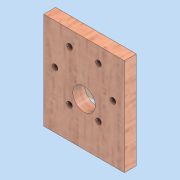
# Autodesk Inventor part: Motor
Saved by Autodesk Inventor 2021 (Build 250183000, 183)
## iProperties
Created: 2021-02-01
Part Number: Motor
Material: Generic
Document SubType Name: Modeling
Designer: garre
Density: 1 g/cm^3
Appearance: Default
Author: garre
Autodesk Inventor part; units mm, degrees
ref_plane "YZ Plane" through (0, 0, 0) normal (1, 0, 0) x (0, 1, 0)
ref_plane "XZ Plane" through (0, 0, 0) normal (0, 1, 0) x (-1, 0, 0)
ref_plane "XY Plane" through (0, 0, 0) normal (0, 0, 1) x (1, 0, 0)
sketch "Sketch1" plane through (0, 0, 0) normal (0, 0, 1) x (1, 0, 0)
  point P0 (0, 0)
ref_plane "Work Plane1" through (0, 0, 0) normal (0, 0, 1) x (1, 0, 0)
sketch "Sketch5" plane through (0, 0, 0) normal (0, 0, 1) x (1, 0, 0)
  circle A0 centre (-15.5, 0) radius 1.5
  circle A1 centre (0, 0) radius 18.4 projected
  line L0 (-18.4, 0) -> (18.4, 0)
  line L1 (-1.5961, -18.3306) -> (-1.5961, -18.3306)
  line L2 (0, 18.4) -> (0, -18.4)
  circle A2 centre (0, -7) radius 6
  circle A3 centre (15.5, 0) radius 1.5
  circle A4 centre (0, 0) radius 15.5
  line L3 (-11.863, 20.6629) -> (9.25, -15.9059)
  circle A5 centre (0, 0) radius 18.4 projected
  line L4 (-9.2, -15.9349) -> (9.2, 15.9349)
  circle A6 centre (7.8, -13.3944) radius 1.5
  circle A7 centre (7.75, 13.4234) radius 1.5
  circle A8 centre (-7.75, -13.4234) radius 1.5
  circle A9 centre (-7.6999, 13.4522) radius 1.5
  line L5 (0, 0) -> (-21.575, 0)
  line L6 (-21.575, 0) -> (-21.575, 21.575)
  line L7 (-21.575, 21.575) -> (21.575, 21.575)
  line L8 (21.575, 21.575) -> (21.575, -30.3062)
  line L9 (21.575, -30.3062) -> (-21.575, -30.3062)
  line L10 (-21.575, -30.3062) -> (-21.575, 21.575)
  point P0 (7.75, 13.4234)
  point P1 (7.8, -13.3944)
  point P2 (-0.5944, -1.0295)
  point P3 (0, 0.1156)
  point P4 (0.6654, -1.037)
  point P5 (0.0667, 0)
  dimension "d10" = 3
  dimension "d11" = 12
  dimension "d12" = 7
  dimension "d15" = 3
  dimension "d16" = 31
  dimension "d17" = 2.9
  dimension "d19" = 60
  dimension "d20" = 60
  dimension "d21" = 3
  dimension "d22" = 3
  dimension "d23" = 3
  dimension "d24" = 3
  dimension "d33" = 21.575
  dimension "d34" = 43.15
  dimension "d35" = 30.3062
  dimension "d36" = 21.575
  constraints: 22 end point, 11 point on circle, 8 centre point, 7 point on line, 4 coincident, 3 midpoint, 2 horizontal, 2 parallel, 2 perpendicular, 1 tangent, 1 vertical, 4 other
  measures "d10" diameter of A0
  measures "d11" diameter of A2
  measures "d12" vertical distance of A2.centre A0.centre
  measures "d15" diameter of A3
  measures "d16" distance of A3.centre A0.centre
  measures "d17" distance of L0.start A0.centre
  measures "d19" angle of L0 L3
  measures "d20" angle of L0 L4
  measures "d21" diameter of A6
  measures "d22" diameter of A7
  measures "d23" diameter of A8
  measures "d24" diameter of A9
  measures "d33" distance of L5.start L5.end
  measures "d34" distance of L6.end L7.end
  measures "d35" distance from line of L9 point (0, 0)
  measures "d36" distance from line of L7 point (0, 0)
extrude "Extrusion8" add sketch "Sketch5" along normal blind 6.35 contours L0 L4 A2 A8 A4 A0 | A0 A4 A9 L3 L2 L0 | A0 L0 A1 L3 A9 A4 | A4 A8 L4 A1 L0 A0 | L0 L3 A2 L2 | L2 A2 L4 | L3 L4 A7 A4 A3 L0 | L0 A3 A4 A6 L3 A2 | L3 A9 A4 L2 | L2 A4 A7 L4 L3 | L6 L7 L8 L9 L10 | L3 A1 L2 A4 A9 | L4 A2 L2 A4 A8 | A8 A4 L2 A1 L4 | L2 A1 L4 A7 A4 | A2 L3 A6 A4 L2 | A4 A7 L4 A1 L0 A3 | A3 L0 A1 L3 A6 A4 | A4 A6 L3 A1 L2 picked at (-0.0661, -0.6678)
equation "\"d33\" = MountOffset"
equation "\"d34\" = 2 * MountOffset"
equation "\"d35\" = longMountLength"
equation "\"d36\" = shortMountLength"
equation "\"d37\" = mountDepth"
equation "\"motorDiameter\" = 36.8"
equation "\"mountDepth\" = 6.35"
equation "\"MountOffset\" = 21.575"
equation "\"longMountLength\" = 30.30625"
equation "\"shortMountLength\" = 21.575"
body "Solid2"
